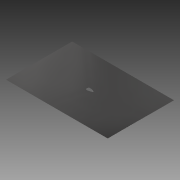
# Autodesk Inventor part: antennal_lobe_sheet_model_v03
Saved by Autodesk Inventor 2015 (Build 190159000, 159)
## iProperties
Created: 2014-11-04
Part Number: antennal_lobe_sheet_model_v03
Material: Stainless Steel AISI 317
Document SubType Name: Sheet Metal
Designer: stephenholtz
Density: 8 g/cm^3
Sheet Metal Rule: Default
Appearance: Semi-Polished
Author: stephenholtz
Autodesk Inventor part; units mm, degrees
ref_plane "YZ Plane" through (0, 0, 0) normal (1, 0, 0) x (0, 1, 0)
ref_plane "XZ Plane" through (0, 0, 0) normal (0, 1, 0) x (-1, 0, 0)
ref_plane "XY Plane" through (0, 0, 0) normal (0, 0, 1) x (1, 0, 0)
sketch "stock_cut_for_holder" plane through (0, 0, 0) normal (0, 1, 0) x (-1, 0, 0)
  line L0 (-12.7, -8.255) -> (12.7, -8.255)
  line L1 (12.7, -8.255) -> (12.7, 8.255)
  line L2 (12.7, 8.255) -> (-12.7, 8.255)
  line L3 (-12.7, 8.255) -> (-12.7, -8.255)
  line L4 (-12.7, -8.255) -> (12.7, 8.255) construction
  line L5 (12.7, -8.255) -> (-12.7, 8.255) construction
  point P0 (0, 0)
  dimension "cut_shim_height" = 25.4
  dimension "cut_shim_width" = 16.51
  measures "cut_shim_height" distance of L2.end L1.end
  measures "cut_shim_width" distance of L0.end L1.end
extrude "Plate1" add sketch "stock_cut_for_holder" along normal blind 0.0254
sketch "mill_path" plane through (0, 0.0254, 0) normal (0, 1, 0) x (1, 0, 0)
  line L0 (12.7, 8.255) -> (12.7, -8.255) projected
  line L1 (-12.7, 8.255) -> (12.7, 8.255) projected
  line L2 (-12.7, -8.255) -> (-12.7, 8.255) projected
  line L3 (12.7, -8.255) -> (-12.7, -8.255) projected
  line L4 (-12.7, 8.255) -> (-12.7, -8.255) projected
  line L5 (-12.7, 0) -> (12.7, 0) construction
  line L6 (12.7, -8.255) -> (12.7, 8.255) projected
  line L7 (0, 0) -> (0, -0.381) construction
  line L8 (0, 0) -> (0, 0.381) construction
  line L9 (-0.4445, 0) -> (-0.4445, -0.4255) construction
  line L10 (-0.4445, 0) -> (-0.4445, 0.4254) construction
  line L11 (0.5842, 0) -> (0.5842, -0.1905) construction
  line L12 (-0.6795, 0) -> (-0.6795, -0.3747) construction
  line L13 (0.5842, 0) -> (0.5842, 0.1905) construction
  line L14 (-0.6795, 0) -> (-0.6795, 0.3746) construction
  line L15 (-0.5398, 0) -> (-0.5397, -0.4001) construction
  line L16 (-0.5398, 0) -> (-0.5398, 0.4) construction
  line L17 (0.5842, 0) -> (0.5842, 0.1905) construction
  line L18 (-0.7747, 0) -> (-0.7747, -0.1778) construction
  line L19 (-0.7747, 0) -> (-0.7747, 0.1778)
  line L20 (0.8382, 0) -> (0.8382, -0.0419) construction
  line L21 (0.8382, 0) -> (0.8382, 0.0419) construction
  spline S0 degree 3 poles (0, -0.381) (0.3656, -0.3096) (0.8827, -0.082) (0.8572, 0) knots 0 0 0 0 1 1 1 1
  spline S1 degree 3 poles (0, 0.381) (0.3656, 0.3096) (0.8827, 0.082) (0.8572, 0) knots 0 0 0 0 1 1 1 1
  line L22 (0, -0.381) -> (-0.4445, -0.4255) construction
  line L23 (-0.4445, -0.4255) -> (-0.5397, -0.4001) construction
  line L24 (-0.5397, -0.4001) -> (-0.6795, -0.3747) construction
  line L25 (-0.6795, -0.3747) -> (-0.7747, -0.1778) construction
  line L26 (-0.7747, -0.1778) -> (-0.7849, 0) construction
  line L27 (-0.7849, 0) -> (-0.7747, 0.1778) construction
  line L28 (-0.7747, 0.1778) -> (-0.6795, 0.3746) construction
  line L29 (-0.6795, 0.3746) -> (-0.5398, 0.4) construction
  line L30 (-0.5398, 0.4) -> (-0.4445, 0.4254) construction
  line L31 (-0.4445, 0.4254) -> (0, 0.381) construction
  spline S2 degree 4 poles (0, -0.381) (-0.4445, -0.4255) (-0.5397, -0.4001) (-0.6795, -0.3747) (-0.7747, -0.1778) (-0.7849, 0) (-0.7747, 0.1778) (-0.6795, 0.3746) (-0.5398, 0.4) (-0.4445, 0.4254) (0, 0.381) knots 1 1 1 1 1 2 3 4 5 6 7 8 8 8 8 8
  dimension "half_mid_thorax_width" = 0.381
  dimension "mid_thorax_to_prescutum" = 0.4445
  dimension "w2" = 0.4254
  dimension "d9" = 0.1905
  dimension "mid_thorax_to_anterior_scutellum" = 0.5842
  dimension "d11" = 0.3746
  dimension "d13" = 0.4001
  dimension "head_thorax" = 0.0953
  dimension "d15" = 0.1397
  dimension "d17" = 0.1778
  dimension "d18" = 0.0953
  dimension "scutellum_taper" = 0.254
  dimension "d20" = 0.0419
  dimension "d21" = 0.0191
  dimension "d22" = 0.0102
  dimension "d24" = 0.3302
  dimension "d25" = 1.6421
  constraints: 30 end point, 9 coincident, 7 vertical, 7 vertical alignment, 2 midpoint, 22 other
  measures "half_mid_thorax_width" distance of L7.start L7.end
  measures "mid_thorax_to_prescutum" distance of L7.start L9.start
  measures "w2" distance of L9.start L9.end
  measures "d9" distance of L11.start L11.end
  measures "mid_thorax_to_anterior_scutellum" distance of L11.start L7.start
  measures "d11" distance of L12.start L12.end
  measures "d13" distance of L15.start L15.end
  measures "head_thorax" distance between parallel lines of L15 L9
  measures "d15" distance between parallel lines of L15 L12
  measures "d17" distance of L18.start L18.end
  measures "d18" distance between parallel lines of L12 L18
  measures "scutellum_taper" distance between parallel lines of L11 L20
  measures "d20" distance of L20.start L20.end
  measures "d21" distance from line of L20 point (0.857, 0)
  measures "d22" distance from line of L18 point (-0.785, 0)
  measures "d24" distance between parallel lines of L19 L10
  measures "d25" distance of point (0.857, 0) point (-0.785, 0)
extrude "milled_hole" cut sketch "mill_path" against normal blind 0.0254 contours S2 S1 S0
fillet "Corner Round1" radius 0.127 1 edges at (0.8572, 0.0127, 0)
equation "\"d26\" = Thickness"
equation "\"BendRadius\" = Thickness"
equation "\"BendReliefWidth\" = Thickness"
equation "\"BendReliefDepth\" = 0.5 * Thickness"
equation "\"CornerReliefSize\" = 4 * Thickness"
equation "\"MinimumRemnant\" = 2 * Thickness"
equation "\"TransitionRadius\" = BendRadius"
equation "\"JacobiRadiusSize\" = BendRadius"
equation "\"GapSize\" = Thickness"
equation "\"d2\" = BendRadius"
equation "\"Thickness\" = 0.0254"
body "Solid1"
